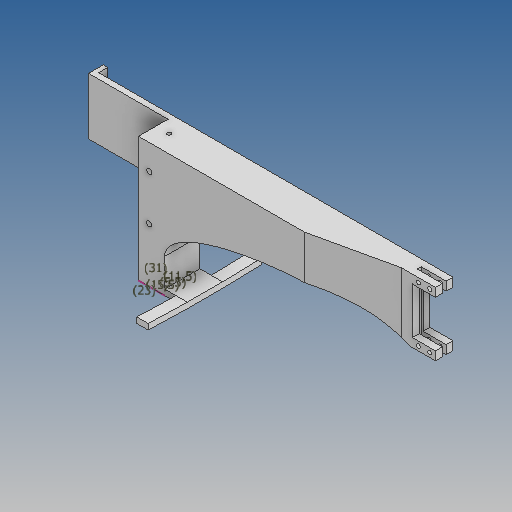
# Autodesk Inventor part: Korpus
Saved by Autodesk Inventor 2026.2 (Build 302298000, 298)
## iProperties
Created: 2025-08-31
Part Number: Korpus
Material: Generisch
Document SubType Name: Modeling
Designer: weyer
Density: 1 g/cm^3
Appearance: Vorgabe
Author: weyer
Autodesk Inventor part; units mm, degrees
ref_plane "YZ Plane" through (0, 0, 0) normal (1, 0, 0) x (0, 1, 0)
ref_plane "XZ Plane" through (0, 0, 0) normal (0, 1, 0) x (-1, 0, 0)
ref_plane "XY Plane" through (0, 0, 0) normal (0, 0, 1) x (1, 0, 0)
sketch "Skizze1" plane through (0, 0, 0) normal (0, 0, 1) x (1, 0, 0)
  line L0 (-9.5, -10.5) -> (7.5, -10.5)
  line L1 (7.5, -10.5) -> (7.5, 10.5)
  line L2 (7.5, 10.5) -> (-9.5, 10.5)
  line L3 (-14.1, 0) -> (18.1, 0) projected
  line L4 (0, -21.7) -> (0, 21.7) projected
  line L5 (-9.5, -10.5) -> (-9.5, -15.5)
  line L6 (-9.5, -15.5) -> (13.5, -15.5)
  line L7 (-9.5, 10.5) -> (-9.5, 15.5)
  line L8 (-9.5, 15.5) -> (13.5, 15.5)
  line L9 (13.5, 15.5) -> (13.5, -15.5)
  point P0 (0, 0)
  dimension "d2" = 21
  dimension "d4" = 7.5
  dimension "d5" = 5
  dimension "d8" = 5
  dimension "d9" = 23
  dimension "d147" = 6
  dimension "d148" = 23
  constraints: 16 end point, 4 perpendicular, 2 vertical, 1 horizontal, 1 other
  measures "d2" distance between parallel lines of L0 L2
  measures "d4" distance between parallel lines of L1 L4
  measures "d5" distance of L0.start L5.end
  measures "d8" distance of L2.end L7.end
  measures "d9" distance of L7.end L8.end
  measures "d147" distance between parallel lines of L1 L9
  measures "d148" distance between parallel lines of L9 L5
extrude "Tower" add sketch "Skizze1" against normal blind 100 contours L0 L4 L6 L5 | L0 L1 L3 L9 L6 L4 | L1 L2 L4 L8 L9 L3 | L2 L7 L8 L4
ref_plane "Arbeitsebene1" through (0, 0, -100) normal (0, 0, -1) x (-1, 0, 0)
sketch "Skizze6" plane through (-9.5, 15.5, 0) normal (0, 1, 0) x (1, 0, 0)
  line L0 (0, 0) -> (23, 0) projected
  line L1 (0, 0) -> (0, -10)
  line L2 (0, -10) -> (228, -10)
  line L3 (23, 0) -> (23, 100) projected
  line L4 (0, -10) -> (246, -10)
  line L5 (246, -10) -> (246, 46)
  line L6 (246, 46) -> (224, 46)
  line L7 (246, 46) -> (268, 46) construction
  line L8 (23, 71.167) -> (23, 0)
  line L9 (0, 0) -> (17, 0) projected
  line L10 (0, 0) -> (0, -12)
  line L11 (246, -12) -> (246, -10)
  spline S0 degree 4 poles (224, 46) (217.2503, 45.4128) (195.5245, 22.479) (125.572, 22.5752) (22.0276, 45.7385) (23, 71.167) knots 0 0 0 0 0 0.374897 1 1 1 1 1
  line L12 (221.3219, 44.8948) -> (192.3718, 31.261) construction
  arc A0 (195.0075, 33.4464) -> (217.9584, 44.255) centre (166.5411, 123.6635) ccw construction
  line L13 (148.8192, 27.3272) -> (94.421, 32.9509) construction
  arc A1 (99.9704, 33.0497) -> (143.4073, 28.5591) centre (158.3015, 384.9585) ccw construction
  line L14 (0, 0) -> (0, 100) projected
  point P0 (9.5, 0)
  point P1 (206.8469, 38.0779)
  point P2 (121.6201, 30.1391)
  point P3 (23, 70.1618)
  dimension "d34" = 10
  dimension "d38" = 246
  dimension "d39" = 56
  dimension "d40" = 180
  dimension "d41" = 22
  constraints: 22 end point, 4 midpoint, 3 point on line, 2 centre point, 2 collinear, 2 perpendicular, 2 point on circle, 2 vertical, 1 horizontal, 6 other
  measures "d34" distance of L0.start L1.end
  measures "d38" distance of L1.end L4.end
  measures "d39" distance of L4.end L5.end
  measures "d40" angle of L6 L7
  measures "d41" distance of L5.end L6.end
extrude "Gripperbogen" add sketch "Skizze6" against normal blind 31 contours L0 L3 S0 L6 L5 L4 L2 L1
sketch "Skizze9" plane through (-9.5, 15.5, 10) normal (0, 0, 1) x (1, 0, 0)
  line L0 (216, -15.5) -> (246, -15.5)
  line L1 (246, 0) -> (246, -31) projected
  line L2 (216, -15.5) -> (246, -15.5) construction
  line L3 (246, -15.5) -> (246, -31)
  line L4 (224, 0) -> (224, -31) projected
  line L5 (246, -9.5) -> (224, -9.5)
  line L6 (224, -9.5) -> (224, -6)
  line L7 (224, -6) -> (246, -6)
  line L8 (246, -6) -> (246, -9.5)
  line L9 (0, 0) -> (246, 0) projected
  line L10 (0, 0) -> (246, 0) projected
  line L11 (0, 0) -> (0, -31) projected
  line L12 (246, -31) -> (0, -31) projected
  line L13 (246, 0) -> (246, -31) projected
  line L14 (216, -15.5) -> (146, -31)
  point P0 (9.5, -15.5)
  point P1 (246, -6)
  point P2 (235, -6)
  dimension "d61" = 3.5
  dimension "d150" = 6
  dimension "d151" = 6
  dimension "d152" = 100
  dimension "d153" = 30
  constraints: 16 end point, 3 point on line, 2 collinear, 2 horizontal, 2 midpoint, 2 parallel, 1 perpendicular
  measures "d61" distance of L5.end L6.end
  measures "d150" distance between parallel lines of L7 L9
  measures "d151" distance between parallel lines of L0 L5
  measures "d152" distance from line of L3 L14.end
  measures "d153" distance from line of L3 L0.start
extrude "Extrusion8" cut sketch "Skizze9" against normal blind 74.5 contours L0 L4 L12 L14 | L0 L1 L12 L4 | L4 L7 L1 L5
sketch "Skizze10" plane through (-9.5, 15.5, -100) normal (0, 1, 0) x (1, 0, 0)
  line L0 (225.7282, -61.6) -> (255.0049, -61.6)
  line L1 (255.0049, -61.6) -> (255.0049, -102.4)
  line L2 (255.0049, -102.4) -> (225.7282, -102.4)
  line L3 (225.7282, -102.4) -> (225.7282, -61.6)
  line L4 (0, -110) -> (246, -110) projected
  line L5 (246, -54) -> (224, -54) projected
  point P0 (9.5, -100)
  dimension "d64" = 7.6
  dimension "d65" = 7.6
  constraints: 8 end point, 2 parallel, 1 horizontal, 1 perpendicular
  measures "d64" distance between parallel lines of L2 L4
  measures "d65" distance between parallel lines of L5 L0
extrude "Extrusion9" cut sketch "Skizze10" against normal blind 74.5
sketch "Skizze12" plane through (0, 0, -100) normal (0, 0, -1) x (-1, 0, 0)
  line L0 (-214.5, 9.5) -> (-236.5, 9.5) projected
  line L1 (-236.5, 15.5) -> (-236.5, 9.5) projected
  line L2 (9.5, 15.5) -> (-236.5, 15.5) projected
  line L3 (9.5, 15.5) -> (9.5, -15.5) projected
  line L4 (-136.5, -15.5) -> (9.5, -15.5) projected
  line L5 (-136.5, -15.5) -> (-206.5, 0) projected
  line L6 (-206.5, 0) -> (-236.5, 0) projected
  line L7 (-236.5, 6) -> (-236.5, 0) projected
  line L8 (-236.5, 6) -> (-214.5, 6) projected
  line L9 (-214.5, 6) -> (-214.5, 9.5) projected
  line L10 (-7.5, 10.5) -> (9.5, 10.5) projected
  line L11 (9.5, 10.5) -> (9.5, 15.5) projected
  line L12 (9.5, 15.5) -> (-13.5, 15.5) projected
  line L13 (-13.5, 15.5) -> (-13.5, -15.5) projected
  line L14 (-13.5, -15.5) -> (9.5, -15.5) projected
  line L15 (9.5, -15.5) -> (9.5, -10.5) projected
  line L16 (9.5, -10.5) -> (-7.5, -10.5) projected
  line L17 (-7.5, -10.5) -> (-7.5, 10.5) projected
  line L18 (-13.5, 15.5) -> (-13.5, -15.5) projected
  line L19 (-13.5, -15.5) -> (9.5, -15.5)
  line L20 (9.5, -15.5) -> (9.5, 15.5)
  line L21 (9.5, 15.5) -> (-13.5, 15.5)
  line L22 (-13.5, 15.5) -> (-13.5, -15.5)
  point P0 (9.5, 25.25)
  point P1 (-13.5, -5.25)
  point P2 (-13.5, 15.5)
  constraints: 8 end point, 2 parallel, 1 horizontal, 1 perpendicular
extrude "Extrusion10" add sketch "Skizze12" against normal blind 10 contours L2 L3 L10 L17 L16 L4 L13 | L3 L16 L17 L10
ref_plane "Arbeitsebene3" through (0, 0, -113.5) normal (0, 0, -1) x (-1, 0, 0)
ref_plane "Arbeitsebene4" through (-9.5, -5.25, -113.5) normal (-1, 0, 0) x (0, 0, 1)
sketch "Skizze18" plane through (0, 0, -90) normal (0, 0, 1) x (1, 0, 0)
  line L0 (7.5, 10.5) -> (7.5, -10.5) projected
  line L1 (-9.5, 10.5) -> (7.5, 10.5) projected
  circle A0 centre (2, 0) radius 2.75
  line L2 (7.5, -10.5) -> (-9.5, -10.5) projected
  line L3 (-9.5, 10.5) -> (-9.5, -10.5) projected
  point P0 (0, 0)
  dimension "d132" = 5.5
  dimension "d154" = 0
  dimension "d155" = 11.5
  dimension "d161" = 21
  dimension "d162" = 17
  constraints: 1 centre point
  measures "d132" diameter of A0
  measures "d154" vertical distance of point (0, 0) A0.centre
  measures "d155" distance from line of L3 A0.centre
  measures "d161" distance between parallel lines of L2 L1
  measures "d162" distance between parallel lines of L0 L3
extrude "Extrusion15" cut sketch "Skizze18" against normal through all contours A0
sketch "Skizze19" plane through (-9.5, -15.5, -100) normal (-1, 0, 0) x (0, 0, 1)
  line L0 (0, 0) -> (0, 31) projected
  line L1 (110, 0) -> (0, 0) projected
  line L2 (110, 31) -> (110, 0) projected
  line L3 (0, 31) -> (110, 31) projected
  line L4 (100, 26) -> (10, 26) projected
  line L5 (100, 26) -> (100, 5) projected
  line L6 (100, 5) -> (10, 5) projected
  line L7 (60, 31) -> (60, 0)
  line L8 (10, 26) -> (10, 5) projected
  line L9 (10, 26) -> (0, 26)
  line L10 (10, 5) -> (0, 5)
  line L11 (100, 26) -> (110, 26)
  line L12 (10, 26) -> (10, 5) projected
  point P0 (100, 15.5)
  point P1 (23.5, 25.5)
  point P2 (23.5, 5)
  point P3 (60, 26)
  point P4 (60, 5)
  point P5 (20, 10.25)
  dimension "d113" = 50
  constraints: 8 end point, 5 point on line, 4 perpendicular, 1 other
  measures "d113" distance between parallel lines of L7 L2
extrude "Extrusion16" add sketch "Skizze19" along normal blind 70 contours L11 L4 L7 L3 L2
sketch "Skizze27" plane through (206.3978, 0, 10) normal (0, -1, 0) x (1, 0, 0)
  line L0 (9.8304, -7.6) -> (30.1022, -7.6) projected
  line L1 (30.1022, 0) -> (30.1022, -7.6) projected
  line L2 (0.1022, 0) -> (30.1022, 0) projected
  line L3 (0.1022, 0) -> (0.1022, -52.845) projected
  line L4 (30.1022, -56) -> (8.1022, -56) projected
  line L5 (30.1022, -48.4) -> (30.1022, -56) projected
  line L6 (30.1022, -48.4) -> (9.8304, -48.4) projected
  line L7 (9.8304, -48.4) -> (9.8304, -7.6) projected
  circle A0 centre (25.1022, -3.8) radius 1.75
  circle A1 centre (15.1022, -3.8) radius 1.75
  line L8 (30.1022, 0) -> (30.1022, -7.6) projected
  circle A2 centre (25.1022, -52.2) radius 1.75
  circle A3 centre (15.1022, -52.2) radius 1.75
  point P0 (-206.3978, -10)
  point P1 (30.1022, -3.8)
  point P2 (28.2249, -52.2)
  point P3 (30.1022, -52.2)
  dimension "d120" = 3.5
  dimension "d121" = 5
  dimension "d122" = 3.5
  dimension "d123" = 10
  dimension "d127" = 3.5
  dimension "d129" = 3.5
  constraints: 5 horizontal alignment, 4 centre point, 2 midpoint, 2 vertical alignment, 1 other
  measures "d120" diameter of A0
  measures "d121" distance from line of A0.centre L1
  measures "d122" diameter of A1
  measures "d123" distance of A1.centre A0.centre
  measures "d127" diameter of A3
  measures "d129" diameter of A2
extrude "Extrusion18" cut sketch "Skizze27" against normal blind 15
sketch "Skizze15" plane through (-9.5, -15.5, -100) normal (0, -1, 0) x (1, 0, 0)
  line L0 (23, 0) -> (0, 0) projected
  line L1 (23, 29.8382) -> (23, 0) projected
  circle A0 centre (9.5, 48) radius 2.25
  circle A1 centre (9.5, 88) radius 2.25
  line L2 (146, 110) -> (0, 110) projected
  line L3 (0, 110) -> (0, 0) projected
  line L4 (146, 71.4914) -> (146, 110) projected
  point P0 (9.5, 100)
  dimension "d138" = 4.5
  dimension "d142" = 4.5
  dimension "d143" = 40
  dimension "d156" = 22
  dimension "d157" = 9.5
  constraints: 2 centre point, 1 vertical alignment, 1 other
  measures "d138" diameter of A0
  measures "d142" diameter of A1
  measures "d143" distance of A1.centre A0.centre
  measures "d156" distance from line of L2 A1.centre
  measures "d157" distance from line of L3 A1.centre
extrude "Extrusion13" cut sketch "Skizze15" against normal blind 100
sketch "Skizze32" plane through (-9.5, -15.5, 10) normal (0, 0, 1) x (1, 0, 0)
  circle A0 centre (11.5, 15.5) radius 2.75 projected
  line L0 (0, 0) -> (0, 31) projected
  line L1 (0, 31) -> (23, 31) projected
  line L2 (23, 31) -> (23, 0) projected
  line L3 (23, 0) -> (0, 0) projected
  circle A1 centre (11.5, 15.5) radius 1.75
  point P0 (9.5, 15.5)
  dimension "d158" = 3.5
  constraints: 1 centre point, 1 coincident
  measures "d158" diameter of A1
extrude "Extrusion20" cut sketch "Skizze32" against normal blind 10 contours A1
sketch "Skizze34" plane through (0, 0, -100) normal (0, 0, -1) x (-1, 0, 0)
  circle A0 centre (-2, 0) radius 2.75 projected
  line L0 (9.5, -15.5) -> (9.5, 15.5) projected
  line L1 (9.5, 15.5) -> (-13.5, 15.5) projected
  line L2 (-13.5, 15.5) -> (-13.5, -15.5) projected
  line L3 (-13.5, -15.5) -> (9.5, -15.5) projected
  point P0 (0, 0)
  dimension "d171" = 23
  dimension "d172" = 31
  dimension "d173" = 15.5
  dimension "d174" = 11.5
  dimension "d175" = 5.5
  measures "d171" distance of L2.end L0.start
  measures "d172" distance of L0.start L0.end
  measures "d173" distance from line of L3 A0.centre
  measures "d174" distance from line of L2 A0.centre
  measures "d175" diameter of A0
sketch "Skizze35" plane through (13.5, -15.5, -100) normal (1, 0, 0) x (0, 0, -1)
  line L0 (-29.8382, 31) -> (0, 31) projected
  line L1 (-29.8382, 0) -> (0, 0) projected
  line L2 (0, 31) -> (0, 0) projected
  line L3 (-29.8382, 31) -> (0, 31) projected
  line L4 (-29.8382, 31) -> (-29.8382, 0) projected
  line L5 (-29.8382, 0) -> (0, 0) projected
  line L6 (0, 31) -> (0, 0) projected
  line L7 (0, 0) -> (-5, 0)
  line L8 (-5, 0) -> (-5, 31)
  line L9 (-5, 31) -> (0, 31)
  line L10 (0, 31) -> (0, 0)
  point P0 (-100, 15.5)
  point P1 (-5, 31)
  point P2 (-5, 0)
  dimension "d176" = 5
  constraints: 8 end point, 2 parallel, 1 horizontal, 1 perpendicular, 1 point on line
  measures "d176" distance of L8.end L9.end
extrude "Extrusion22" add sketch "Skizze35" along normal blind 10 contours L0 L2 L1 L8
sketch "Skizze36" plane through (23.5, -15.5, -100) normal (1, 0, 0) x (0, 0, -1)
  line L0 (-5, 0) -> (0, 0) projected
  line L1 (0, 0) -> (0, 31) projected
  line L2 (0, 31) -> (-5, 31) projected
  line L3 (-5, 31) -> (-5, 0) projected
  arc A0 (-9.879, -89.9986) -> (-9.879, 121.0014) centre (-1120.404, 15.5014) ccw
  line L4 (-5, 15.5) -> (0, 15.5)
  arc A1 (-4.9014, -90.4715) -> (-4.9014, 121.4742) centre (-1120.404, 15.5014) ccw
  line L5 (-5, 15.5) -> (0, 15.5)
  line L6 (-14.7679, -34.5) -> (17.3967, -34.5)
  line L7 (-14.7679, 65.5) -> (14.0644, 65.5)
  point P0 (-100, 15.5)
  point P1 (-0.9951, 65.5)
  point P2 (-6.0001, 65.5)
  point P3 (-4.9867, 31)
  point P4 (-4.9867, 0)
  point P5 (-6.0002, -34.5)
  point P6 (-0.9952, -34.5)
  dimension "d181" = 5
  dimension "d182" = 100
  constraints: 8 end point, 4 point on circle, 3 horizontal, 2 centre point, 2 midpoint, 1 other
  measures "d181" radial gap between concentric circles of A0 A1
  measures "d182" distance between parallel lines of L7 L6
extrude "Extrusion23" add sketch "Skizze36" along normal blind 10
sketch "Skizze37" plane through (214.5, 15.5, -46) normal (0, 1, 0) x (1, 0, 0)
  line L0 (-224, -6) -> (-294, -6) projected
  line L1 (-294, -56) -> (-294, -6) projected
  line L2 (-294, -56) -> (22, -56) projected
  line L3 (-294, -56) -> (-290, -56)
  line L4 (-290, -56) -> (-290, -52)
  line L5 (-290, -52) -> (-294, -52)
  line L6 (-294, -52) -> (-294, -56)
  line L7 (-294, -6) -> (-290, -6)
  line L8 (-290, -6) -> (-290, -10)
  line L9 (-290, -10) -> (-294, -10)
  line L10 (-294, -10) -> (-294, -6)
  point P0 (-214.5, -46)
  point P1 (-294, -54)
  point P2 (-294, -8)
  point P3 (-290, -54)
  point P4 (-290, -8)
  dimension "d185" = 0
  dimension "d186" = 0
  dimension "d187" = 4
  dimension "d188" = 4
  dimension "d189" = 0
  dimension "d190" = 4
  constraints: 16 end point, 4 midpoint, 4 parallel, 2 horizontal, 2 perpendicular, 2 vertical alignment
  measures "d185" distance between parallel lines of L1 L6
  measures "d186" distance between parallel lines of L2 L3
  measures "d187" distance between parallel lines of L5 L3
  measures "d188" distance between parallel lines of L4 L6
  measures "d189" distance between parallel lines of L0 L7
  measures "d190" distance between parallel lines of L7 L9
extrude "Extrusion24" add sketch "Skizze37" along normal blind 8
sketch "Skizze38" plane through (-75.5, 15.5, 6) normal (0, 0, -1) x (-1, 0, 0)
  line L0 (4, 0) -> (4, 8) projected
  line L1 (0, 8) -> (4, 8) projected
  line L2 (0, 0) -> (0, 8) projected
  line L3 (0, 8) -> (4, 8)
  line L4 (4, 8) -> (4, 4)
  line L5 (4, 4) -> (0, 4)
  line L6 (0, 4) -> (0, 8)
  point P0 (-75.5, -15.5)
  point P1 (0, 4)
  dimension "d193" = 4
  constraints: 8 end point, 2 parallel, 1 horizontal, 1 midpoint, 1 perpendicular
  measures "d193" distance of L3.end L4.end
extrude "Extrusion25" add sketch "Skizze38" along normal blind 4
sketch "Skizze39" plane through (-79.5, 15.5, -36) normal (0, 0, 1) x (1, 0, 0)
  line L0 (4, 0) -> (4, 8) projected
  line L1 (0, 8) -> (4, 8) projected
  line L2 (0, 0) -> (0, 8) projected
  line L3 (0, 4) -> (0, 8) projected
  line L4 (0, 8) -> (4, 8) projected
  line L5 (4, 8) -> (4, 4) projected
  line L6 (4, 4) -> (0, 4) projected
  point P0 (79.5, -15.5)
extrude "Extrusion26" add sketch "Skizze39" along normal blind 4
